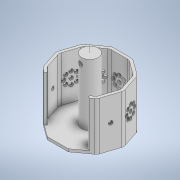
# Autodesk Inventor part: holder-10
Saved by Autodesk Inventor 2020 (Build 240168000, 168)
## iProperties
Created: 2020-02-16
Part Number: holder-10
Material: Generic
Document SubType Name: Modeling
Designer: Ball
Density: 1 g/cm^3
Appearance: Default
Author: Ball
Autodesk Inventor part; units mm, degrees
ref_plane "YZ Plane" through (0, 0, 0) normal (1, 0, 0) x (0, 1, 0)
ref_plane "XZ Plane" through (0, 0, 0) normal (0, 1, 0) x (-1, 0, 0)
sketch "Sketch1" plane through (0, 0, 0) normal (0, 1, 0) x (-1, 0, 0)
  line L0 (53.4143, 0) -> (43.2131, -31.3961)
  line L1 (43.2131, -31.3961) -> (16.5059, -50.8)
  line L2 (16.5059, -50.8) -> (-16.5059, -50.8)
  line L3 (-16.5059, -50.8) -> (-43.2131, -31.3961)
  line L4 (-43.2131, -31.3961) -> (-53.4143, 0)
  line L5 (-53.4143, 0) -> (-43.2131, 31.3961)
  line L6 (-43.2131, 31.3961) -> (-16.5059, 50.8)
  line L7 (-16.5059, 50.8) -> (16.5059, 50.8)
  line L8 (16.5059, 50.8) -> (43.2131, 31.3961)
  line L9 (43.2131, 31.3961) -> (53.4143, 0)
  point P0 (0, 0)
  point P1 (0, 0)
  dimension "d0" = 50.8
  constraints: 20 end point, 1 coincident, 21 other
  measures "d0" distance from line of L7 point (0, 0)
extrude "Extrusion1" add sketch "Sketch1" along normal blind 76.2
sketch "Sketch2" plane through (0, 76.2, 0) normal (0, 1, 0) x (1, 0, 0)
  line L0 (-48.9275, 0) -> (-39.5832, 28.7589)
  line L1 (-39.5832, 28.7589) -> (-15.1194, 46.5328)
  line L2 (-15.1194, 46.5328) -> (15.1194, 46.5328)
  line L3 (15.1194, 46.5328) -> (39.5832, 28.7589)
  line L4 (39.5832, 28.7589) -> (48.9275, 0)
  line L5 (48.9275, 0) -> (39.5832, -28.7589)
  line L6 (39.5832, -28.7589) -> (33.02, -33.5273)
  line L7 (-33.02, -33.5273) -> (-39.5832, -28.7589)
  line L8 (-39.5832, -28.7589) -> (-48.9275, 0)
  line L9 (-43.2131, 31.3961) -> (-53.4143, 0) projected
  line L10 (-3.2307, -59.865) -> (3.2307, -59.865)
  line L11 (0, -59.865) -> (-33.02, -59.865)
  line L12 (-33.02, -59.865) -> (33.02, -59.865)
  line L13 (33.02, -59.865) -> (33.02, -33.5273)
  line L14 (-33.02, -59.865) -> (-33.02, -33.5273)
  point P0 (0, 0)
  point P1 (0, 0)
  dimension "d3" = 4.2672
  dimension "d90" = 33.02
  dimension "d91" = 66.04
  constraints: 28 end point, 4 point on line, 1 coincident, 1 midpoint, 1 parallel, 1 perpendicular, 16 other
  measures "d3" distance between parallel lines of L0 L9
  measures "d90" distance of L11.start L11.end
  measures "d91" distance of L11.end L12.end
extrude "Extrusion2" cut sketch "Sketch2" against normal blind 71.9328
fillet "Fillet1" radius 1.905 4 edges at (-33.02, 40.2336, 38.8018) (-33.02, 40.2336, 33.5273) (33.02, 40.2336, 38.8018) (33.02, 40.2336, 33.5273)
fillet "Fillet2" radius 8.89 7 edges at (-48.9275, 40.2336, 0) (-15.1194, 40.2336, -46.5328) (15.1194, 40.2336, -46.5328) (-39.5832, 40.2336, -28.7589) (-39.5832, 40.2336, 28.7589) (39.5832, 40.2336, -28.7589) (48.9275, 40.2336, 0)
fillet "Fillet3" radius 8.89 8 edges at (43.2131, 38.1, 31.3961) (53.4143, 38.1, 0) (43.2131, 38.1, -31.3961) (16.5059, 38.1, -50.8) (-16.5059, 38.1, -50.8) (-43.2131, 38.1, -31.3961) (-53.4143, 38.1, 0) (-43.2131, 38.1, 31.3961)
sketch "Sketch5" plane through (52.5217, 0, 2.7472) normal (0.9511, 0, 0.309) x (0.309, 0, -0.9511)
  circle A0 centre (-13.6174, 38.1) radius 2.921
  line L0 (-27.2348, 76.2) -> (0, 76.2) projected
  point P0 (-13.6174, 0)
  dimension "d27" = 5.842
  dimension "d28" = 38.1
  constraints: 1 centre point
  measures "d27" diameter of A0
  measures "d28" distance from line of L0 A0.centre
extrude "Extrusion5" cut sketch "Sketch5" against normal through all
sketch "Sketch6" plane through (-44.1057, 0, 28.649) normal (-0.9511, 0, 0.309) x (0.309, 0, 0.9511)
  circle A0 centre (-13.6174, 38.1) radius 2.921
  point P0 (-13.6174, 0)
  dimension "d31" = 5.842
  constraints: 1 centre point
  measures "d31" diameter of A0
extrude "Extrusion6" cut sketch "Sketch6" against normal through all
sketch "Sketch8" plane through (13.6174, 0, -50.8) normal (0, 0, -1) x (-1, 0, 0)
  circle A0 centre (13.6174, 38.1) radius 2.921
  line L0 (0, 76.2) -> (27.2348, 76.2) projected
  circle A1 centre (4.1432, 38.1) radius 2.921
  circle A2 centre (6.9181, 31.4007) radius 2.921
  circle A3 centre (13.6174, 28.6258) radius 2.921
  circle A4 centre (20.3167, 31.4007) radius 2.921
  circle A5 centre (23.0916, 38.1) radius 2.921
  circle A6 centre (20.3167, 44.7993) radius 2.921
  circle A7 centre (13.6174, 47.5742) radius 2.921
  circle A8 centre (6.9181, 44.7993) radius 2.921
  point P0 (13.6174, 0)
  dimension "d34" = 5.842
  dimension "d35" = 38.1
  dimension "d57" = 5.842
  dimension "d58" = 9.4742
  dimension "d61" = 360
  constraints: 9 centre point, 17 other
  measures "d34" diameter of A0
  measures "d35" distance from line of L0 A0.centre
  measures "d57" diameter of A1
  measures "d58" distance of A1.centre A0.centre
extrude "Extrusion7" cut sketch "Sketch8" against normal blind 25.4
sketch "Sketch9" plane through (-40.8762, 0, -33.094) normal (-0.5878, 0, -0.809) x (-0.809, 0, 0.5878)
  line L0 (0, 76.2) -> (0, 0) projected
  line L1 (-27.2348, 0) -> (-27.2348, 76.2) projected
  circle A0 centre (-13.6144, 38.1) radius 2.921
  circle A1 centre (-4.1402, 38.1) radius 2.921
  circle A2 centre (-6.9151, 44.7993) radius 2.921
  circle A3 centre (-13.6144, 47.5742) radius 2.921
  circle A4 centre (-20.3137, 44.7993) radius 2.921
  circle A5 centre (-23.0886, 38.1) radius 2.921
  circle A6 centre (-20.3137, 31.4007) radius 2.921
  circle A7 centre (-13.6144, 28.6258) radius 2.921
  circle A8 centre (-6.9151, 31.4007) radius 2.921
  point P0 (-13.6174, 0)
  dimension "d39" = 5.842
  dimension "d40" = 13.6144
  dimension "d51" = 5.842
  dimension "d52" = 9.4742
  dimension "d55" = 360
  constraints: 9 centre point, 17 other
  measures "d39" diameter of A0
  measures "d40" distance from line of L0 A0.centre
  measures "d51" diameter of A1
  measures "d52" distance of A1.centre A0.centre
extrude "Extrusion8" cut sketch "Sketch9" against normal blind 25.4
sketch "Sketch10" plane through (18.8428, 0, -49.1022) normal (0.5878, 0, -0.809) x (-0.809, 0, -0.5878)
  circle A0 centre (-13.6204, 38.1) radius 2.921
  line L0 (-27.2348, 0) -> (0, 0) projected
  line L1 (-27.2348, 0) -> (-27.2348, 76.2) projected
  circle A1 centre (-4.1462, 38.1) radius 2.921
  circle A2 centre (-6.9211, 44.7993) radius 2.921
  circle A3 centre (-13.6204, 47.5742) radius 2.921
  circle A4 centre (-20.3196, 44.7993) radius 2.921
  circle A5 centre (-23.0946, 38.1) radius 2.921
  circle A6 centre (-20.3196, 31.4007) radius 2.921
  circle A7 centre (-13.6204, 28.6258) radius 2.921
  circle A8 centre (-6.9211, 31.4007) radius 2.921
  point P0 (-13.6174, 0)
  dimension "d43" = 5.842
  dimension "d44" = 38.1
  dimension "d45" = 13.6144
  dimension "d63" = 5.842
  dimension "d64" = 9.4742
  dimension "d67" = 360
  constraints: 9 centre point, 17 other
  measures "d43" diameter of A0
  measures "d44" distance from line of L0 A0.centre
  measures "d45" distance from line of L1 A0.centre
  measures "d63" diameter of A1
  measures "d64" distance of A0.centre A1.centre
extrude "Extrusion9" cut sketch "Sketch10" against normal blind 25.4
sketch "Sketch11" plane through (0, 4.2672, 0) normal (0, 1, 0) x (1, 0, 0)
  circle A0 centre (0, 0) radius 12.954
  dimension "d48" = 25.908
  constraints: 1 centre point, 1 coincident
  measures "d48" diameter of A0
extrude "Extrusion10" add sketch "Sketch11" along normal blind 97.3328
sketch "Sketch12" plane through (44.1057, 0, -28.649) normal (0.9511, 0, -0.309) x (-0.309, 0, -0.9511)
  circle A0 centre (-4.1432, 38.1) radius 2.921
  circle A1 centre (-13.6174, 38.1) radius 2.921 projected
  circle A2 centre (-6.9181, 44.7993) radius 2.921
  circle A3 centre (-13.6174, 47.5742) radius 2.921
  circle A4 centre (-20.3167, 44.7993) radius 2.921
  circle A5 centre (-23.0916, 38.1) radius 2.921
  circle A6 centre (-20.3167, 31.4007) radius 2.921
  circle A7 centre (-13.6174, 28.6258) radius 2.921
  circle A8 centre (-6.9181, 31.4007) radius 2.921
  point P0 (-13.6174, 0)
  dimension "d69" = 5.842
  dimension "d70" = 9.4742
  dimension "d73" = 360
  constraints: 8 centre point, 17 other
  measures "d69" diameter of A0
  measures "d70" distance of A1.centre A0.centre
extrude "Extrusion11" cut sketch "Sketch12" against normal blind 25.4 contours A0 | A2 | A3 | A4 | A5 | A6 | A7 | A8
sketch "Sketch13" plane through (-52.5217, 0, -2.7472) normal (-0.9511, 0, -0.309) x (-0.309, 0, 0.9511)
  circle A0 centre (-4.1432, 38.1) radius 2.921
  circle A1 centre (-13.6174, 38.1) radius 2.921 projected
  circle A2 centre (-6.9181, 44.7993) radius 2.921
  circle A3 centre (-13.6174, 47.5742) radius 2.921
  circle A4 centre (-20.3167, 44.7993) radius 2.921
  circle A5 centre (-23.0916, 38.1) radius 2.921
  circle A6 centre (-20.3167, 31.4007) radius 2.921
  circle A7 centre (-13.6174, 28.6258) radius 2.921
  circle A8 centre (-6.9181, 31.4007) radius 2.921
  point P0 (-13.6174, 0)
  dimension "d77" = 5.842
  dimension "d78" = 9.4742
  dimension "d81" = 360
  constraints: 8 centre point, 17 other
  measures "d77" diameter of A0
  measures "d78" distance of A1.centre A0.centre
extrude "Extrusion12" cut sketch "Sketch13" against normal blind 25.4 contours A0 | A2 | A3 | A4 | A5 | A6 | A7 | A8
ref_plane "Work Plane1" through (0, 4.2672, 0) normal (-0.2017, 0, 0.9794) x (0, -1, 0)
sketch "Sketch14" plane through (0, 4.2672, 0) normal (-0.2017, 0, 0.9794) x (0, -1, 0)
  circle A0 centre (-87.1728, 0) radius 3.81
  line L0 (-97.3328, 12.954) -> (-97.3328, -12.954) projected
  point P0 (4.2672, 0)
  dimension "d85" = 7.62
  dimension "d86" = 10.16
  constraints: 1 centre point
  measures "d85" diameter of A0
  measures "d86" distance from line of L0 A0.centre
extrude "Extrusion13" cut sketch "Sketch14" against normal through all both and the other way through all
body "Solid1"
